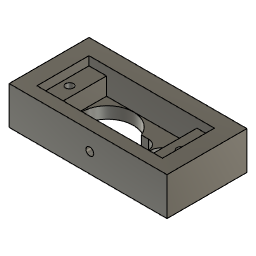
Robocrab Base v6 (Autodesk Fusion 360 design; units mm, degrees)
Autodesk Fusion 360 part; units mm, degrees
sketch "Base" plane through (0, 0, 0) normal (0, 0, 1) x (1, 0, 0)
  line L0 (21.2961, 35) -> (61.7961, 35)
  line L1 (61.7961, 35) -> (61.7961, 14.5)
  line L2 (61.7961, 14.5) -> (21.2961, 14.5)
  line L3 (21.2961, 14.5) -> (21.2961, 35)
  dimension "d1" = 40.5
  dimension "d2" = 20.5
  constraint horizontal L0
  constraint vertical L1
  constraint horizontal L2
  constraint vertical L3
  measures "d1" distance of L1 L3
  measures "d2" distance of L0 L2
extrude "Extrude1" add sketch "Base" along normal blind 9.75 makes body 1
sketch "Hollow 1" plane through (0, 0, 9.75) normal (0, 0, 1) x (-1, 0, 0)
  line L0 (-21.2961, -14.5) -> (-61.7961, -14.5)
  line L1 (-61.7961, -14.5) -> (-61.7961, -35)
  line L2 (-61.7961, -35) -> (-21.2961, -35)
  line L3 (-21.2961, -35) -> (-21.2961, -14.5)
  line L4 (-25.3461, -30.925) -> (-57.5461, -30.925)
  line L5 (-57.5461, -30.925) -> (-57.5461, -17.575)
  line L6 (-57.5461, -17.575) -> (-25.3461, -17.575)
  line L7 (-25.3461, -17.575) -> (-25.3461, -30.925)
  line L8 (-21.2961, -35) -> (-61.7961, -35)
  line L9 (-61.7961, -14.5) -> (-21.2961, -14.5)
  line L10 (-21.2961, -14.5) -> (-21.2961, -35)
  line L11 (-61.7961, -35) -> (-61.7961, -14.5)
  dimension "d5" = 13.35
  dimension "d6" = 32.2
  dimension "d7" = 3.075
  dimension "d8" = 3.4
  dimension "d9" = 20.5
  dimension "d10" = 40.5
  dimension "d11" = 4.05
  constraint horizontal L4
  constraint vertical L5
  constraint horizontal L6
  constraint vertical L7
  measures "d5" distance of L4 L6
  measures "d6" distance of L5 L7
  measures "d7" distance of L0 L6
  measures "d9" distance of L8 L9
  measures "d10" distance of L10 L11
  measures "d11" distance of L7 L10
extrude "Extrude2" cut sketch "Hollow 1" against normal blind 2.25 contours L4 L5 L6 L7 bodies 1
sketch "Hollow 2" plane through (0, 0, 7.5) normal (0, 0, 1) x (-1, 0, 0)
  line L0 (-25.3461, -17.575) -> (-57.5461, -17.575)
  line L1 (-57.5461, -17.575) -> (-57.5461, -30.925)
  line L2 (-57.5461, -30.925) -> (-25.3461, -30.925)
  line L3 (-25.3461, -30.925) -> (-25.3461, -17.575)
  line L4 (-29.8461, -30.925) -> (-53.0461, -30.925)
  line L5 (-53.0461, -30.925) -> (-53.0461, -17.575)
  line L6 (-53.0461, -17.575) -> (-29.8461, -17.575)
  line L7 (-29.8461, -17.575) -> (-29.8461, -30.925)
  dimension "d19" = 4.5
  dimension "d20" = 4.5
  constraint horizontal L4
  constraint vertical L5
  constraint horizontal L6
  constraint vertical L7
  constraint coincident L0 L5.end
  constraint coincident L2 L4.start
  measures "d19" distance of L3 L7
  measures "d20" distance of L1 L5
extrude "Extrude3" cut sketch "Hollow 2" against normal blind 4.5 contours L0 L2 L4 L5 L6 L7 bodies 1
sketch "Holes" plane through (0, 0, 3) normal (0, 0, 1) x (-1, 0, 0)
  line L0 (-29.8461, -17.575) -> (-53.0461, -17.575)
  line L1 (-53.0461, -17.575) -> (-53.0461, -30.925)
  line L2 (-53.0461, -30.925) -> (-29.8461, -30.925)
  line L3 (-29.8461, -30.925) -> (-29.8461, -17.575)
  circle A0 centre (-36.7961, -24.235) radius 6.665
  line L4 (-42.954, -26.785) -> (-42.954, -21.685)
  line L5 (-42.954, -26.785) -> (-44.779, -26.785)
  line L6 (-47.229, -24.335) -> (-47.229, -24.135)
  line L7 (-44.779, -21.685) -> (-42.954, -21.685)
  arc A1 (-47.229, -24.335) -> (-44.779, -26.785) centre (-44.779, -24.335) ccw
  arc A2 (-44.779, -21.685) -> (-47.229, -24.135) centre (-44.779, -24.135) ccw
  point P0 (-47.229, -26.785)
  point P1 (-47.229, -21.685)
  dimension "d23" = 13.33
  dimension "d24" = 6.95
  dimension "d25" = 6.66
  dimension "d29" = 5.1
  dimension "d30" = 5.1
  dimension "d32" = 2.45
  constraint coincident A0 L4.start
  constraint coincident A0 L4.end
  constraint perpendicular L2 L4
  constraint horizontal L5
  constraint vertical L6
  constraint horizontal L7
  constraint coincident P0 L5
  constraint coincident P0 L6
  constraint tangent L5 A1
  constraint tangent L6 A1
  constraint coincident P1 L6
  constraint coincident P1 L7
  constraint tangent L6 A2
  constraint tangent L7 A2
  constraint equal A1 A2
  measures "d23" diameter of A0
  measures "d24" distance of L3 A0.centre
  measures "d25" distance of L0 A0.centre
  measures "d29" distance of L4.start L4.end
  measures "d30" distance of P0 P1
  measures "d32" radius of A1
extrude "Extrude4" cut sketch "Holes" against normal through all contours A0 L4 bodies 1
extrude "Extrude5" cut sketch "Holes" against normal through all contours A0 L5 L6 L7 A1 A2 bodies 1
extrude "Extrude6" add sketch "Holes" against normal through all of body 1 separate body contours L0 A0 L4 | L0 A0 makes body 2
extrude "Extrude7" cut sketch "Holes" against normal through all contours L0 A0 L4 | L0 A0 bodies 2
extrude "Extrude8" cut sketch "Holes" against normal through all contours L0 A0 L4 bodies 1
sketch "Holes 2" plane through (0, 0, 0) normal (0, 0, -1) x (1, 0, 0)
  arc A0 (42.954, -21.685) -> (37.0542, -17.575) centre (36.7961, -24.235) ccw
  line L0 (42.954, -21.685) -> (44.779, -21.685)
  arc A1 (47.229, -24.135) -> (44.779, -21.685) centre (44.779, -24.135) ccw
  line L1 (47.229, -24.135) -> (47.229, -24.335)
  arc A2 (44.779, -26.785) -> (47.229, -24.335) centre (44.779, -24.335) ccw
  line L2 (44.779, -26.785) -> (42.954, -26.785)
  arc A3 (36.538, -17.575) -> (42.954, -26.785) centre (36.7961, -24.235) ccw
  line L3 (36.538, -17.575) -> (37.0542, -17.575)
  line L4 (61.7961, -14.5) -> (21.2961, -14.5)
  line L5 (21.2961, -14.5) -> (21.2961, -35)
  line L6 (21.2961, -35) -> (61.7961, -35)
  line L7 (61.7961, -35) -> (61.7961, -14.5)
  circle A4 centre (50.862, -24.2941) radius 3.38
  circle A5 centre (55.7961, -24.0242) radius 1
  circle A6 centre (27.2961, -24) radius 1
  dimension "d40" = 2
  dimension "d41" = 6
  dimension "d42" = 2
  dimension "d43" = 6
  measures "d40" diameter of A5
  measures "d41" distance of L7 A5.centre
  measures "d42" diameter of A6
  measures "d43" distance of L5 A6.centre
extrude "Extrude9" cut sketch "Holes 2" against normal through all contours A6 bodies 1
extrude "Extrude10" cut sketch "Holes 2" against normal through all contours A5 bodies 1
extrude "Extrude11" cut sketch "Holes 2" against normal blind 5 contours A4 bodies 1
sketch "Attachments" plane through (0, 35, 0) normal (0, 1, 0) x (-1, 0, 0)
  line L0 (-61.7961, 0) -> (-21.2961, 0)
  line L1 (-21.2961, 0) -> (-21.2961, 9.75)
  line L2 (-21.2961, 9.75) -> (-61.7961, 9.75)
  line L3 (-61.7961, 9.75) -> (-61.7961, 0)
  circle A0 centre (-55.7961, 5) radius 1
  circle A1 centre (-27.2961, 5) radius 1
  dimension "d48" = 2
  dimension "d49" = 6
  dimension "d50" = 4.75
  dimension "d51" = 2
  dimension "d52" = 4.75
  dimension "d53" = 6
  measures "d48" diameter of A0
  measures "d49" distance of L3 A0.centre
  measures "d50" distance of L2 A0.centre
  measures "d51" diameter of A1
  measures "d52" distance of L2 A1.centre
  measures "d53" distance of L1 A1.centre
extrude "Extrude12" add sketch "Attachments" against normal blind 3.75 contours A1 bodies 1 2
extrude "Extrude13" add sketch "Attachments" against normal blind 3.75 contours A0 bodies 1
extrude "Extrude14" cut sketch "Attachments" against normal blind 3.75 contours A1 bodies 1
extrude "Extrude15" cut sketch "Attachments" against normal blind 3.75 contours A0 bodies 1
sketch "Attachments 2" plane through (0, 14.5, 0) normal (0, -1, 0) x (1, 0, 0)
  line L0 (21.2961, 0) -> (61.7961, 0)
  line L1 (61.7961, 0) -> (61.7961, 9.75)
  line L2 (61.7961, 9.75) -> (21.2961, 9.75)
  line L3 (21.2961, 9.75) -> (21.2961, 0)
  circle A0 centre (41.9961, 5) radius 1
  dimension "d62" = 2
  dimension "d63" = 4.75
  dimension "d64" = 20.7
  dimension "d66" = 19.803
  measures "d62" diameter of A0
  measures "d63" distance of L2 A0.centre
  measures "d64" distance of L3 A0.centre
extrude "Extrude16" cut sketch "Attachments 2" against normal blind 3.5 contours A0 bodies 1
named bodies: "Base"
